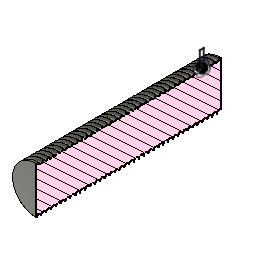
Rope thread (Autodesk Fusion 360 design; units mm, degrees)
Autodesk Fusion 360 part; units mm, degrees
sketch "Sketch1" plane through (0, 0, 0) normal (0, 1, 0) x (1, 0, 0)
  circle A0 centre (0, 0) radius 73
  dimension "d1" = 146
  constraint coincident A0.centre origin
  measures "d1" diameter of A0
extrude "Extrude1" add sketch "Sketch1" along normal blind 575
coil "CoilPrimitive1" cut diameter 146 section circle size 14.2 on centre turns 37.72966 pitch 15.24 right hand placed x (-1, 0, 0) y (0, 0, -1) z (0, -1, 0) at (0, 575, 0)
sketch "Sketch3" plane through (0, 0, 0) normal (1, 0, 0) x (0, 1, 0)
  spline S0 degree 3 poles (524.95, 73) (524.95, 72.5077) (524.8988, 72.0167) (524.6956, 71.0533) (524.5442, 70.5834) (523.9721, 69.2872) (523.4371, 68.5224) (522.1042, 67.241) (521.3189, 66.7365) (519.5993, 66.057) (518.6813, 65.8885) (516.8324, 65.9127) (515.9191, 66.1053) (514.2179, 66.8297) (513.4461, 67.3546) (512.1473, 68.6706) (511.6326, 69.4492) (510.9306, 71.1598) (510.75, 72.0755) (510.75, 73) knots -2.23689 -2.23689 -2.23689 -2.23689 -2.089197 -2.089197 -1.941503 -1.941503 -1.664145 -1.664145 -1.386788 -1.386788 -1.10943 -1.10943 -0.832073 -0.832073 -0.554715 -0.554715 -0.277358 -0.277358 0 0 0 0
  arc A0 (510.75, 73) -> (524.95, 73) centre (517.85, 73) ccw
  line L0 (523.95, 71.9046) -> (523.95, 123)
  line L1 (523.95, 123) -> (511.95, 123)
  line L2 (511.95, 123) -> (511.95, 71.9046)
  arc A1 (511.95, 71.9046) -> (523.95, 71.9046) centre (517.95, 71.9046) ccw
  line L3 (517.85, 73) -> (517.95, 73) construction
  line L4 (517.95, 73) -> (517.95, 71.9046) construction
  line L5 (517.95, 71.9046) -> (517.85, 73) construction
  line L6 (511.1342, 65.9) -> (524.9633, 65.9)
  dimension "d9" = 14.2
  dimension "d10" = 12
  dimension "d16" = 50
  dimension "d19" = 7.1
  dimension "d20" = 7
  constraint tangent A0 A1
  constraint tangent L0 A1
  constraint perpendicular L0 L1
  constraint perpendicular L1 L2
  constraint tangent L2 A1
  constraint horizontal L1
  constraint coincident A0.centre L3.start
  constraint horizontal L3
  constraint coincident A1.centre L4.end
  constraint perpendicular L3 L4
  constraint horizontal L6
  constraint tangent A0 L6
  measures "d9" diameter of A0
  measures "d10" diameter of A1
  measures "d16" distance of A0.centre L1
  measures "d19" distance of S0.start L6
  measures "d20" distance of S0.start A1.centre
